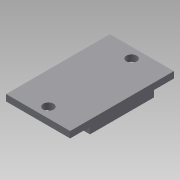
# Autodesk Inventor part: peltier and mount
Saved by Autodesk Inventor 2015 (Build 190159000, 159)
## iProperties
Created: 2015-05-21
Part Number: peltier and mount
Material: Generic
Document SubType Name: Modeling
Designer: Joe Sheldon
Density: 1 g/cm^3
Appearance: Default
Author: Joe Sheldon
Autodesk Inventor part; units mm, degrees
ref_plane "YZ Plane" through (0, 0, 0) normal (1, 0, 0) x (0, 1, 0)
ref_plane "XZ Plane" through (0, 0, 0) normal (0, 1, 0) x (-1, 0, 0)
ref_plane "XY Plane" through (0, 0, 0) normal (0, 0, 1) x (1, 0, 0)
sketch "Sketch1" plane through (0, 0, 0) normal (0, 1, 0) x (-1, 0, 0)
  line L0 (0, 0) -> (38.1, 0)
  line L1 (38.1, 0) -> (38.1, -38.1)
  line L2 (38.1, -38.1) -> (0, -38.1)
  line L3 (0, -38.1) -> (0, 0)
  dimension "d0" = 38.1
  dimension "d1" = 38.1
  constraints: 8 end point, 2 parallel, 1 horizontal, 1 perpendicular
  measures "d0" distance of L1.end L2.end
  measures "d1" distance of L0.end L1.end
extrude "Extrusion1" add sketch "Sketch1" along normal blind 3.81
sketch "Sketch2" plane through (0, 3.81, 0) normal (0, 1, 0) x (1, 0, 0)
  line L0 (-38.1, 0) -> (0, 0) projected
  line L1 (0, 0) -> (0, 38.1) projected
  line L2 (0, 38.1) -> (-38.1, 38.1) projected
  line L3 (-38.1, 38.1) -> (-38.1, 0) projected
  line L4 (-38.1, 0) -> (0, 0)
  line L5 (0, 0) -> (0, -11.8097)
  line L6 (0, -11.8097) -> (-38.1, -11.8097)
  line L7 (-38.1, -11.8097) -> (-38.1, 0)
  line L8 (-38.1, 38.1) -> (0, 38.1)
  line L9 (0, 38.1) -> (0, 49.9227)
  line L10 (0, 49.9227) -> (-38.1, 49.9227)
  line L11 (-38.1, 49.9227) -> (-38.1, 38.1)
  constraints: 16 end point, 4 parallel, 2 horizontal, 2 perpendicular, 1 point on line
extrude "Extrusion2" add sketch "Sketch2" along normal blind 3.81
sketch "Sketch3" plane through (0, 7.62, 0) normal (0, 1, 0) x (1, 0, 0)
  line L0 (-38.1, -11.8097) -> (0, -11.8097) projected
  line L1 (-19.05, -11.8097) -> (-19.05, -5.7137)
  line L2 (0, 49.9227) -> (-38.1, 49.9227) projected
  line L3 (-19.05, 49.9227) -> (-19.05, 43.8267)
  circle A0 centre (-19.05, -5.7137) radius 3.048
  circle A1 centre (-19.05, 43.8267) radius 3.048
  point P0 (0, 0)
  dimension "d6" = 6.096
  dimension "d7" = 6.096
  dimension "d8" = 6.096
  constraints: 4 end point, 2 centre point, 2 coincident, 2 midpoint, 2 vertical
  measures "d6" distance of L1.start L1.end
  measures "d7" distance of L3.start L3.end
  measures "d8" diameter of A0
extrude "Extrusion3" cut sketch "Sketch3" against normal blind 3.81
body "Solid1"
